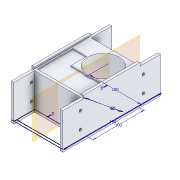
# Autodesk Inventor part: MiddlePart
Saved by Autodesk Inventor 2020.3 (Build 243373010, 373A)
## iProperties
Created: 2020-12-04
Part Number: MiddlePart
Material: Generic
Document SubType Name: Modeling
Designer: Yusuf
Mass: 275.041 g
Surface Area: 1350.9 cm^2
Volume: 275.041 cm^3
Density: 1 g/cm^3
Appearance: Default
Author: Yusuf
Autodesk Inventor part; units mm, degrees
ref_plane "YZ Plane" through (0, 0, 0) normal (1, 0, 0) x (0, 1, 0)
ref_plane "XZ Plane" through (0, 0, 0) normal (0, 1, 0) x (-1, 0, 0)
ref_plane "XY Plane" through (0, 0, 0) normal (0, 0, 1) x (1, 0, 0)
sketch "Sketch1" plane through (0, 0, 0) normal (0, 1, 0) x (-1, 0, 0)
  line L0 (0, 0) -> (0, -190)
  line L1 (0, -190) -> (100, -190)
  line L2 (100, -190) -> (100, 0)
  line L3 (100, 0) -> (0, 0)
  line L4 (95, -5) -> (95, -185)
  line L5 (95, -185) -> (5, -185)
  line L6 (5, -185) -> (5, -5)
  line L7 (5, -5) -> (95, -5)
  line L8 (95, -5) -> (95, 0)
  line L9 (95, -185) -> (95, -190)
  line L10 (5, -185) -> (5, -190)
  line L11 (5, -5) -> (5, 0)
  line L12 (100, -45) -> (0, -45)
  line L13 (0, -45) -> (0, -145)
  line L14 (0, -145) -> (100, -145)
  line L15 (100, -145) -> (100, -45)
  line L16 (100, -40) -> (0, -40)
  line L17 (100, -150) -> (0, -150)
  point P0 (100, -95)
  point P1 (100, -95)
  point P2 (5, -150)
  point P3 (95, -150)
  point P4 (95, -40)
  point P5 (5, -40)
  point P6 (95, -145)
  point P7 (5, -145)
  point P8 (5, -45)
  point P9 (95, -45)
  dimension "d0" = 190
  dimension "d1" = 100
  dimension "d2" = 100
  dimension "d3" = 5
  dimension "d4" = 5
  constraints: 36 end point, 10 point on line, 9 perpendicular, 2 horizontal, 2 midpoint, 2 parallel, 1 coincident, 1 vertical
  measures "d0" distance of L0.start L0.end
  measures "d1" distance of L0.end L1.end
  measures "d2" distance of L13.end L12.end
  measures "d3" distance between parallel lines of L16 L12
  measures "d4" distance between parallel lines of L17 L14
extrude "Extrusion1" add sketch "Sketch1" along normal blind 65 contours L3 L11 L6 L16 L0 | L16 L6 L12 L0 | L12 L6 L14 L0 | L3 L2 L16 L4 L8 | L14 L6 L17 L0 | L16 L2 L12 L4 | L17 L6 L10 L1 L0 | L12 L2 L14 L4 | L14 L2 L17 L4 | L17 L2 L1 L9 L4
extrude "Extrusion2" add sketch "Sketch1" against normal blind 5 contours L3 L11 L6 L16 L0 | L16 L6 L12 L0 | L12 L6 L14 L0 | L16 L4 L12 L6 | L3 L2 L16 L4 L8 | L14 L6 L17 L0 | L12 L4 L14 L6 | L16 L2 L12 L4 | L17 L6 L10 L1 L0 | L14 L4 L17 L6 | L12 L2 L14 L4 | L14 L2 L17 L4 | L17 L2 L1 L9 L4
extrude "Extrusion3" add sketch "Sketch1" along normal blind 65 contours L14 L4 L17 L6
extrude "Extrusion5" add sketch "Sketch1" along normal blind 65 contours L16 L4 L12 L6
sketch "Sketch2" plane through (0, 0, 0) normal (0, 1, 0) x (1, 0, 0)
  circle A0 centre (-35.6617, 114.4032) radius 30.5
  circle A1 centre (-35.6617, 114.4032) radius 32.5
  point P0 (0, 0)
  dimension "d11" = 61
  dimension "d12" = 65
  constraints: 2 centre point, 1 coincident
  measures "d11" diameter of A0
  measures "d12" diameter of A1
extrude "Extrusion4" add sketch "Sketch2" along normal blind 65
sketch "Sketch3" plane through (-5, 0, -103.6278) normal (-1, 0, 0) x (0, 0, 1)
  line L0 (-41.3722, 65) -> (-21.5507, 65) projected
  line L1 (58.6278, 0) -> (58.6278, 65) projected
  line L2 (-41.3722, 65) -> (58.6278, 65)
  line L3 (58.6278, 65) -> (58.6278, 62)
  line L4 (58.6278, 62) -> (-41.3722, 62)
  line L5 (-41.3722, 62) -> (-41.3722, 65)
  point P0 (103.6278, 0)
  dimension "d17" = 3
  constraints: 8 end point, 2 parallel, 1 horizontal, 1 perpendicular, 1 point on line
  measures "d17" distance of L2.end L3.end
extrude "Extrusion6" add sketch "Sketch3" along normal up to surface (90 mm away)
extrude "Extrusion7" cut sketch "Sketch2" along normal blind 66.5 contours A0
sketch "Sketch4" plane through (0, 65, 0) normal (0, 1, 0) x (1, 0, 0)
  line L0 (-95, 145) -> (-95, 45) projected
  line L1 (-5, 45) -> (-5, 103.6278) projected
  line L2 (-95, 45) -> (-5, 45)
  line L3 (-5, 45) -> (-5, 83.6142)
  line L4 (-5, 83.6142) -> (-95, 83.6142)
  line L5 (-95, 83.6142) -> (-95, 45)
  arc A0 (-46.6201, 145) -> (-5, 103.6278) centre (-35.6617, 114.4032) ccw projected
  line L6 (-95, 83.6142) -> (-68.1617, 83.6142)
  line L7 (-68.1617, 83.6142) -> (-68.1617, 114.4032)
  line L8 (-68.1617, 114.4032) -> (-95, 114.4032)
  line L9 (-95, 114.4032) -> (-95, 83.6142)
  point P0 (0, 0)
  point P1 (-25.2556, 83.6142)
  point P2 (-46.0678, 83.6142)
  constraints: 16 end point, 4 parallel, 2 horizontal, 2 perpendicular, 1 point on circle, 1 point on line
extrude "Extrusion8" cut sketch "Sketch4" against normal blind 2 contours L8 L7 L4 L0 | L4 A0 L1 L2 L0
sketch "Sketch5" plane through (0, 65, 0) normal (1, 0, 0) x (0, 0, -1)
  circle A0 centre (33.7554, -16.723) radius 5.5293
  circle A1 centre (33.7554, -48.723) radius 5.535
  circle A2 centre (156.2446, -16.723) radius 5.926
  circle A3 centre (156.2446, -48.723) radius 6.0534
  line L0 (33.7554, -16.723) -> (33.7554, -48.723)
  line L1 (33.7554, -16.723) -> (156.2446, -16.723)
  line L2 (0, 0) -> (190, 0) projected
  line L3 (0, -70) -> (0, 0) projected
  line L4 (0, 0) -> (190, 0)
  point P0 (0, -65)
  point P1 (95, -16.723)
  point P2 (33.7554, -32.723)
  point P3 (95, 0)
  dimension "d24" = 16.723
  dimension "d25" = 32
  constraints: 6 end point, 4 centre point, 3 midpoint, 3 vertical alignment, 2 horizontal alignment, 1 perpendicular
  measures "d24" distance from line of L2 L0.start
  measures "d25" distance of L0.end L0.start
hole "Hole1" at (0, 48.277, -33.7554) at (0, 16.277, -33.7554) at (0, 16.277, -156.2446) at (0, 48.277, -156.2446) direction (-1, 0, 0) diameter 4.917 depth 17.1 thread size "M6x1" class "6H" standard "ANSI Metric M Profile"
ref_plane "Work Plane1" through (-50, 65, 0) normal (1, 0, 0) x (0, 0, -1)
mirror "Mirror1" about plane through (-50, 65, 0) normal (1, 0, 0) of "Hole1"
sketch "Sketch6" plane through (0, 65, 0) normal (0, 1, 0) x (1, 0, 0)
  line L0 (-95, 150) -> (-95, 190) projected
  line L1 (-95, 150) -> (-100, 150)
  line L2 (-100, 190) -> (-100, 0) projected
  line L3 (-95, 40) -> (-5, 40) projected
  line L4 (-95, 40) -> (-100, 40)
  line L5 (-100, 150) -> (-95, 150)
  line L6 (-95, 150) -> (-95, 40)
  line L7 (-95, 40) -> (-100, 40)
  line L8 (-100, 40) -> (-100, 150)
  line L9 (0, 0) -> (0, 190) projected
  line L10 (-5, 150) -> (0, 150)
  line L11 (0, 150) -> (0, 40)
  line L12 (0, 40) -> (-5, 40)
  line L13 (-5, 40) -> (-5, 150)
  constraints: 20 end point, 4 parallel, 3 horizontal, 3 point on line, 2 perpendicular, 1 collinear
extrude "Extrusion9" add sketch "Sketch6" along normal blind 6
sketch "Sketch7" plane through (-100, 65, -40) normal (0, 0, 1) x (1, 0, 0)
  line L0 (5, 0) -> (5, 6) projected
  line L1 (5, 4) -> (5, 0)
  line L2 (5, 0) -> (2, 0)
  line L3 (2, 0) -> (2, 4)
  line L4 (2, 4) -> (5, 4)
  line L5 (94.9938, 4) -> (97.9938, 4)
  line L6 (97.9938, 4) -> (97.9938, 0)
  line L7 (97.9938, 0) -> (94.9938, 0)
  line L8 (94.9938, 0) -> (94.9938, 4)
  line L9 (5, 0) -> (5, 6) projected
  line L10 (0, 0) -> (5, 0) projected
  line L11 (95, 0) -> (100, 0) projected
  point P0 (100, -65)
  dimension "d35" = 4
  dimension "d36" = 3
  dimension "d37" = 3
  dimension "d38" = 4
  dimension "d39" = 0
  dimension "d40" = 0
  constraints: 16 end point, 3 perpendicular, 2 horizontal, 2 parallel, 2 point on line
  measures "d35" distance of L1.start L1.end
  measures "d36" distance of L1.end L2.end
  measures "d37" distance of L6.end L7.end
  measures "d38" distance of L5.end L6.end
  measures "d39" distance between parallel lines of L10 L2
  measures "d40" distance between parallel lines of L11 L7
extrude "Extrusion10" cut sketch "Sketch7" against normal up to surface (110 mm away)
body "Solid1"
